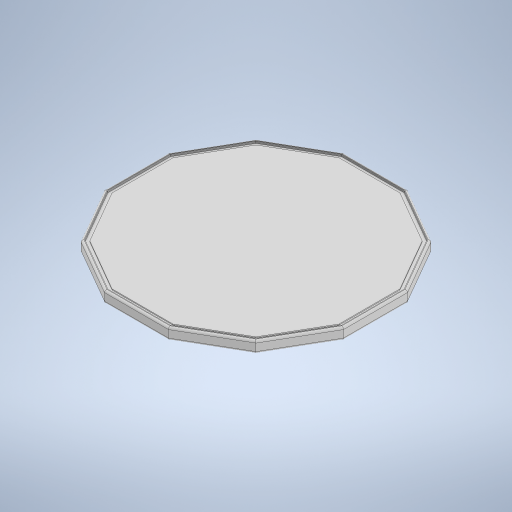
# Autodesk Inventor part: (x2)_POSPA_Large_Bottom
Saved by Autodesk Inventor 2024 (Build 280153000, 153)
## iProperties
Created: 2023-12-08
Part Number: (x2)_POSPA_Large_Bottom
Material: 일반
Document SubType Name: Modeling
Designer: jsw
Density: 1 g/cm^3
Appearance: 기본값
Author: jsw
Autodesk Inventor part; units mm, degrees
ref_plane "YZ Plane" through (0, 0, 0) normal (1, 0, 0) x (0, 1, 0)
ref_plane "XZ Plane" through (0, 0, 0) normal (0, 1, 0) x (-1, 0, 0)
ref_plane "XY Plane" through (0, 0, 0) normal (0, 0, 1) x (1, 0, 0)
sketch "스케치1" plane through (0, 0, 0) normal (0, 1, 0) x (-1, 0, 0)
  line L0 (-49.8892, 49.8892) -> (-18.2607, 68.1499)
  line L1 (-18.2607, 68.1499) -> (18.2607, 68.1499)
  line L2 (18.2607, 68.1499) -> (49.8892, 49.8892)
  line L3 (49.8892, 49.8892) -> (68.1499, 18.2607)
  line L4 (68.1499, 18.2607) -> (68.1499, -18.2607)
  line L5 (68.1499, -18.2607) -> (49.8892, -49.8892)
  line L6 (49.8892, -49.8892) -> (18.2607, -68.1499)
  line L7 (18.2607, -68.1499) -> (-18.2607, -68.1499)
  line L8 (-18.2607, -68.1499) -> (-49.8892, -49.8892)
  line L9 (-49.8892, -49.8892) -> (-68.1499, -18.2607)
  line L10 (-68.1499, -18.2607) -> (-68.1499, 18.2607)
  line L11 (-68.1499, 18.2607) -> (-49.8892, 49.8892)
  line L12 (71.3499, -19.1182) -> (52.2318, -52.2318)
  line L13 (52.2318, -52.2318) -> (19.1182, -71.3499)
  line L14 (19.1182, -71.3499) -> (-19.1182, -71.3499)
  line L15 (-19.1182, -71.3499) -> (-52.2318, -52.2318)
  line L16 (-52.2318, -52.2318) -> (-71.3499, -19.1182)
  line L17 (-71.3499, -19.1182) -> (-71.3499, 19.1182)
  line L18 (-71.3499, 19.1182) -> (-52.2318, 52.2318)
  line L19 (-52.2318, 52.2318) -> (-19.1182, 71.3499)
  line L20 (-19.1182, 71.3499) -> (19.1182, 71.3499)
  line L21 (19.1182, 71.3499) -> (52.2318, 52.2318)
  line L22 (52.2318, 52.2318) -> (71.3499, 19.1182)
  line L23 (71.3499, 19.1182) -> (71.3499, -19.1182)
  point P0 (0, 0)
  point P1 (0, 0)
  point P2 (0, 0)
  dimension "d0" = 141.108
  dimension "d1" = 3.2
  constraints: 48 end point, 2 coincident, 2 horizontal, 50 other
  measures "d0" distance of L8.end L2.end
  measures "d1" distance between parallel lines of L3 L22
extrude "돌출1" add sketch "스케치1" along normal blind 6.8 contours L0 L1 L2 L3 L4 L5 L6 L7 L8 L9 L10 L11 | L12 L13 L14 L15 L16 L17 L18 L19 L20 L21 L22 L23
sketch "스케치2" plane through (0, 6.8, 0) normal (0, 1, 0) x (1, 0, 0)
  line L0 (-18.6894, 69.7499) -> (18.6894, 69.7499)
  line L1 (18.6894, 69.7499) -> (51.0605, 51.0605)
  line L2 (51.0605, 51.0605) -> (69.7499, 18.6894)
  line L3 (69.7499, 18.6894) -> (69.7499, -18.6894)
  line L4 (69.7499, -18.6894) -> (51.0605, -51.0605)
  line L5 (51.0605, -51.0605) -> (18.6894, -69.7499)
  line L6 (18.6894, -69.7499) -> (-18.6894, -69.7499)
  line L7 (-18.6894, -69.7499) -> (-51.0605, -51.0605)
  line L8 (-51.0605, -51.0605) -> (-69.7499, -18.6894)
  line L9 (-69.7499, -18.6894) -> (-69.7499, 18.6894)
  line L10 (-69.7499, 18.6894) -> (-51.0605, 51.0605)
  line L11 (-51.0605, 51.0605) -> (-18.6894, 69.7499)
  line L12 (-71.3499, 19.1182) -> (-71.3499, -19.1182) projected
  line L13 (18.1535, -67.7499) -> (-18.1535, -67.7499)
  line L14 (-18.1535, -67.7499) -> (-49.5964, -49.5964)
  line L15 (-49.5964, -49.5964) -> (-67.7499, -18.1535)
  line L16 (-67.7499, -18.1535) -> (-67.7499, 18.1535)
  line L17 (-67.7499, 18.1535) -> (-49.5964, 49.5964)
  line L18 (-49.5964, 49.5964) -> (-18.1535, 67.7499)
  line L19 (-18.1535, 67.7499) -> (18.1535, 67.7499)
  line L20 (18.1535, 67.7499) -> (49.5964, 49.5964)
  line L21 (49.5964, 49.5964) -> (67.7499, 18.1535)
  line L22 (67.7499, 18.1535) -> (67.7499, -18.1535)
  line L23 (67.7499, -18.1535) -> (49.5964, -49.5964)
  line L24 (49.5964, -49.5964) -> (18.1535, -67.7499)
  point P0 (0, 0)
  point P1 (0, 0)
  point P2 (0, 0)
  dimension "d4" = 1.6
  dimension "d5" = 2
  constraints: 48 end point, 2 coincident, 2 horizontal, 50 other
  measures "d4" distance between parallel lines of L9 L12
  measures "d5" distance between parallel lines of L16 L9
extrude "돌출2" cut sketch "스케치2" against normal blind 1.2
sketch "스케치5" plane through (0, 6.8, 0) normal (0, 1, 0) x (1, 0, 0)
  line L0 (-49.5964, -49.5964) -> (-18.1535, -67.7499) projected
  line L1 (-18.1535, -67.7499) -> (18.1535, -67.7499) projected
  line L2 (18.1535, -67.7499) -> (49.5964, -49.5964) projected
  line L3 (49.5964, -49.5964) -> (67.7499, -18.1535) projected
  line L4 (67.7499, -18.1535) -> (67.7499, 18.1535) projected
  line L5 (67.7499, 18.1535) -> (49.5964, 49.5964) projected
  line L6 (49.5964, 49.5964) -> (18.1535, 67.7499) projected
  line L7 (18.1535, 67.7499) -> (-18.1535, 67.7499) projected
  line L8 (-18.1535, 67.7499) -> (-49.5964, 49.5964) projected
  line L9 (-49.5964, 49.5964) -> (-67.7499, 18.1535) projected
  line L10 (-67.7499, 18.1535) -> (-67.7499, -18.1535) projected
  line L11 (-67.7499, -18.1535) -> (-49.5964, -49.5964) projected
  point P0 (0, 0)
extrude "돌출5" cut sketch "스케치5" against normal blind 0.6
fillet "모깎기1" radius 1.2 24 edges at (61.7909, 0, 35.675) (61.7909, 6.8, 35.675) (71.3499, 6.8, 0) (71.3499, 0, 0) (61.7909, 6.8, -35.675) (61.7909, 0, -35.675) (35.675, 6.8, -61.7909) (35.675, 0, -61.7909) (0, 0, -71.3499) (0, 6.8, -71.3499) (-35.675, 6.8, -61.7909) (-35.675, 0, -61.7909) (-61.7909, 0, -35.675) (-61.7909, 6.8, -35.675) (-71.3499, 0, 0) (-71.3499, 6.8, 0) (-61.7909, 0, 35.675) (-61.7909, 6.8, 35.675) (-35.675, 0, 61.7909) (-35.675, 6.8, 61.7909) (0, 0, 71.3499) (0, 6.8, 71.3499) (35.675, 0, 61.7909) (35.675, 6.8, 61.7909)
sketch "스케치7" plane through (0, 0, 0) normal (0, -1, 0) x (1, 0, 0)
  line L0 (10, -7.5) -> (-10, -7.5)
  line L1 (-10, -7.5) -> (-10, -2.5)
  line L2 (-10, -2.5) -> (10, -2.5)
  line L3 (10, -2.5) -> (10, -7.5)
  line L4 (10, -7.5) -> (-10, -2.5) construction
  line L5 (-10, -7.5) -> (10, -2.5) construction
  line L6 (0, 0) -> (-24.3026, 0)
  line L7 (10, 7.5) -> (-10, 7.5)
  line L8 (-10, 7.5) -> (-10, 2.5)
  line L9 (-10, 2.5) -> (10, 2.5)
  line L10 (10, 2.5) -> (10, 7.5)
  line L11 (10, 7.5) -> (-10, 2.5) construction
  line L12 (-10, 7.5) -> (10, 2.5) construction
  point P0 (0, -5)
  point P1 (0, 5)
  dimension "d26" = 20
  dimension "d27" = 5
  dimension "d28" = 2.5
  constraints: 26 end point, 5 symmetric about line, 2 horizontal, 2 midpoint, 2 parallel, 1 perpendicular, 1 vertical alignment
  measures "d26" distance of L0.start L0.end
  measures "d27" distance of L0.end L1.end
  measures "d28" distance from line of L2 L6.start
extrude "돌출7" add sketch "스케치7" along normal blind 10
sketch "스케치8" plane through (-10, 0, 7.5) normal (0, 0, 1) x (1, 0, 0)
  circle A0 centre (15, -5) radius 1.25
  line L0 (-8.7966, 0) -> (28.7966, 0) projected
  line L1 (20, 0) -> (20, -10) projected
  line L2 (20, -10) -> (0, -10) projected
  line L3 (10, -10) -> (10, 0)
  circle A1 centre (5, -5) radius 1.25
  point P0 (20, -5)
  dimension "d31" = 2.5
  dimension "d32" = 5
  dimension "d33" = 5
  constraints: 2 centre point, 2 end point, 2 midpoint, 1 perpendicular, 1 symmetric about line, 1 other
  measures "d31" diameter of A0
  measures "d32" distance from line of A0.centre L0
  measures "d33" distance of point (20, -5) A0.centre
extrude "돌출8" cut sketch "스케치8" against normal up to surface (15 mm away) contours A0 | A1
